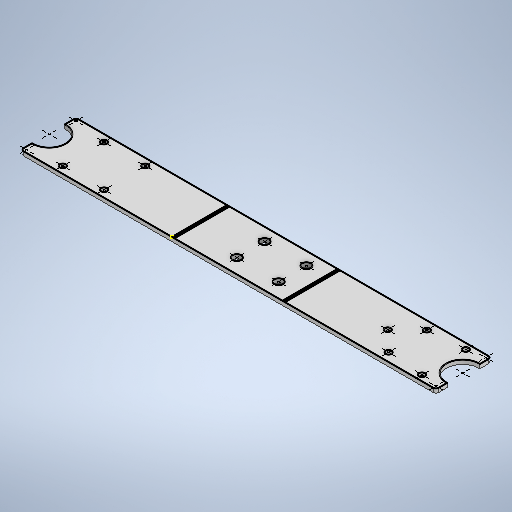
# Autodesk Inventor part: axis_16_top_frame
Saved by Autodesk Inventor 2026.1 (Build 301233000, 233)
## iProperties
Created: 2025-08-15
Part Number: axis_16_top_frame
Material: Generic
Document SubType Name: Modeling
Designer: LG
Density: 1 g/cm^3
Appearance: Default
Author: LG
Autodesk Inventor part; units mm, degrees
ref_plane "YZ Plane" through (0, 0, 0) normal (1, 0, 0) x (0, 1, 0)
ref_plane "XZ Plane" through (0, 0, 0) normal (0, 1, 0) x (-1, 0, 0)
ref_plane "XY Plane" through (0, 0, 0) normal (0, 0, 1) x (1, 0, 0)
sketch "Sketch1" plane through (0, 0, 0) normal (0, 1, 0) x (-1, 0, 0)
  line L0 (-0.4496, -20.14) -> (-0.4496, 0)
  line L1 (-40.8289, 0) -> (-40.8289, -20.14)
  circle A0 centre (-18.3893, -15.45) radius 1.55
  circle A1 centre (-18.3893, -5.31) radius 1.55
  circle A2 centre (-33.6893, -15.45) radius 1.55
  circle A3 centre (-33.6893, -5.31) radius 1.55
  circle A4 centre (27.33, -17.595) radius 1.05
  circle A5 centre (27.33, -2.545) radius 1.05
  circle A6 centre (42.43, -17.595) radius 1.05
  circle A7 centre (42.43, -2.545) radius 1.05
  circle A8 centre (-89.3086, -18.07) radius 1.05
  circle A9 centre (-89.3086, -2.07) radius 1.05
  circle A10 centre (-76.0886, -17.07) radius 1.05
  circle A11 centre (-76.0886, -3.07) radius 1.05
  circle A12 centre (-68.7886, -10.07) radius 1.05
  arc A13 (-96.4686, -19.14) -> (-95.4686, -20.14) centre (-95.4686, -19.14) ccw
  line L2 (-96.4686, -19.14) -> (-96.4686, -16.0644)
  line L3 (54.19, -20.14) -> (-95.4686, -20.14)
  arc A14 (54.19, -20.14) -> (55.19, -19.14) centre (54.19, -19.14) ccw
  line L4 (55.19, -16.0644) -> (55.19, -19.14)
  arc A15 (55.19, -4.0756) -> (55.19, -16.0644) centre (54.93, -10.07) ccw
  line L5 (55.19, -1) -> (55.19, -4.0756)
  arc A16 (55.19, -1) -> (54.19, 0) centre (54.19, -1) ccw
  line L6 (-95.4686, 0) -> (54.19, 0)
  arc A17 (-95.4686, 0) -> (-96.4686, -1) centre (-95.4686, -1) ccw
  line L7 (-96.4686, -4.0756) -> (-96.4686, -1)
  arc A18 (-96.4686, -16.0644) -> (-96.4686, -4.0756) centre (-96.2086, -10.07) ccw
  line L8 (-41.2786, -20.14) -> (-41.2786, 0)
  line L9 (-40.3793, 0) -> (-40.3793, -20.14)
  line L10 (-0.8993, -20.14) -> (-0.8993, 0)
  line L11 (0, 0) -> (0, -20.14)
  constraints: 24 end point, 19 centre point, 15 equal radius, 12 point on circle, 12 point on line, 10 tangent, 10 vertical, 8 parallel, 2 horizontal, 2 perpendicular, 1 collinear, 63 other
extrude "Extrusion1" add sketch "Sketch1" against normal blind 1.5
body "Solid1"
